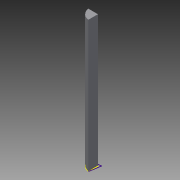
# Autodesk Inventor part: styroFoamMandrel
Saved by Autodesk Inventor 2014 (Build 180170000, 170)
## iProperties
Created: 2014-02-10
Part Number: styroFoamMandrel
Material: Generic
Document SubType Name: Modeling
Designer: clang
Density: 1 g/cm^3
Appearance: Default
Author: clang
Autodesk Inventor part; units mm, degrees
ref_plane "YZ Plane" through (0, 0, 0) normal (1, 0, 0) x (0, 1, 0)
ref_plane "XZ Plane" through (0, 0, 0) normal (0, 1, 0) x (-1, 0, 0)
ref_plane "XY Plane" through (0, 0, 0) normal (0, 0, 1) x (1, 0, 0)
sketch "Sketch1" plane through (0, 0, 0) normal (0, 1, 0) x (-1, 0, 0)
  arc A0 (105.8221, 15.9999) -> (16.0001, 105.822) centre (0, 0) ccw
  line L0 (16.0001, 16.0002) -> (105.8221, 15.9999)
  line L1 (16.0001, 105.822) -> (16.0001, 16.0002)
  arc A1 (105.8221, 15.9999) -> (16.0001, 105.822) centre (0, 0) ccw
  line L2 (16.0001, 16.0002) -> (105.8221, 15.9999)
  line L3 (16.0001, 105.822) -> (16.0001, 16.0002)
  line L4 (16.0001, 105.822) -> (0, 0)
  line L5 (0, 0) -> (105.8221, 15.9999)
  dimension "d2" = 180
  constraints: 12 end point, 4 point on circle, 2 centre point, 1 coincident, 8 other
extrude "Extrusion1" add sketch "Sketch1" along normal blind 1219.2 contours L0 L1 A0
sketch "Sketch2" plane through (0, 0, 0) normal (0, -1, 0) x (1, 0, 0)
  arc A0 (-16.0001, 105.822) -> (-105.8221, 15.9999) centre (0, 0) ccw projected
  line L0 (-16.0001, 16.0002) -> (-105.8221, 15.9999) projected
  line L1 (-16.0001, 105.822) -> (-16.0001, 16.0002) projected
  line L2 (-16.0001, 105.822) -> (0, 0)
  line L3 (0, 0) -> (-105.8221, 15.9999)
  constraints: 4 end point
body "Solid1"
